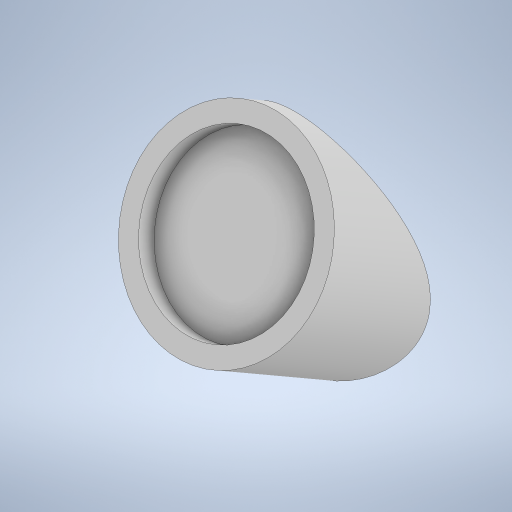
# Autodesk Inventor part: 1'' copper pipe 60 deg mount
Saved by Autodesk Inventor 2024.2 (Build 282272000, 272)
## iProperties
Created: 2024-03-22
Part Number: 1'' copper pipe 60 deg mount
Material: Generic
Document SubType Name: Modeling
Designer: ellix
Density: 1 g/cm^3
Appearance: Default
Author: ellix
Autodesk Inventor part; units mm, degrees
ref_plane "YZ Plane" through (0, 0, 0) normal (1, 0, 0) x (0, 1, 0)
ref_plane "XZ Plane" through (0, 0, 0) normal (0, 1, 0) x (-1, 0, 0)
ref_plane "XY Plane" through (0, 0, 0) normal (0, 0, 1) x (1, 0, 0)
sketch "Sketch1" plane through (0, 0, 0) normal (1, 0, 0) x (0, 1, 0)
  line L0 (22.9037, 13.0375) -> (-26.2512, 13.0375)
  line L1 (-26.2512, 13.0375) -> (-26.2512, -17.8825)
  line L2 (-26.2512, -17.8825) -> (22.9037, -17.8825)
  line L3 (22.9037, -17.8825) -> (22.9037, 13.0375)
  line L4 (-27.7512, 14.5375) -> (24.4037, 14.5375)
  line L5 (24.4037, 14.5375) -> (24.4037, -19.3825)
  line L6 (24.4037, -19.3825) -> (-27.7512, -19.3825)
  line L7 (-27.7512, -19.3825) -> (-27.7512, 14.5375)
  line L8 (14.8755, 31.453) -> (106.1225, 31.453) construction
  line L9 (5.1094, 14.5375) -> (-10.0461, 23.2875)
  line L10 (-10.0461, 23.2875) -> (-9.0461, 25.0195)
  line L11 (-9.0461, 25.0195) -> (-10.7781, 26.0195)
  line L12 (-10.7781, 26.0195) -> (-17.4073, 14.5375)
  line L13 (24.4037, -2.4225) -> (-27.7512, -2.4225)
  point P0 (0, 0)
  point P1 (22.9037, -2.4225)
  point P2 (-26.2512, -2.4225)
  dimension "d0" = 30.92
  dimension "d1" = 1.5
  dimension "d3" = 17.5
  dimension "d4" = 2
  dimension "d5" = 2
  constraints: 28 end point, 4 parallel, 3 horizontal, 3 perpendicular, 2 midpoint, 2 point on line, 3 other
  measures "d0" distance of L2.end L0.start
  measures "d1" distance between parallel lines of L0 L4
  measures "d3" distance of L9.start L9.end
  measures "d4" distance of L9.end L10.end
  measures "d5" distance of L10.end L11.end
ref_plane "Work Plane1" through (0, -10.7781, 26.0195) normal (0, -0.5, -0.8660254) x (1, 0, 0)
sketch "Sketch2" plane through (0, -10.7781, 26.0195) normal (0, -0.5, -0.8660254) x (1, 0, 0)
  line L0 (0, -19.5) -> (0, -2) projected
  circle A0 centre (0, -10.75) radius 8.75
  circle A1 centre (0, -10.75) radius 10.75
  point P0 (0, -22.3439)
  point P1 (0, 0)
  constraints: 2 vertical alignment, 1 coincident, 1 midpoint, 4 other
extrude "Extrusion1" add sketch "Sketch2" along normal blind 19 contours A0 L0 | L0 A0 | A1
extrude "Extrusion2" cut sketch "Sketch2" along normal blind 2 contours A0 L0 | L0 A0
revolve "Revolution1" add sketch "Sketch1" angle 360 about axis through (0, 24.4037, -2.4225) along (0, -1, 0) contours L0 L1 L13 L7 L4 L5 L3
sketch "Sketch3" plane through (0, 24.4037, -2.4225) normal (0, 1, 0) x (1, 0, 0)
  circle A0 centre (0, 0) radius 15.46 projected
  circle A1 centre (0, 0) radius 16.96 projected
  point P0 (0, -2.4225)
extrude "Extrusion3" cut sketch "Sketch3" against normal blind 127.25 contours A0
sketch "Sketch4" plane through (0, 0, 0) normal (1, 0, 0) x (0, 1, 0)
  line L0 (24.4037, 14.5375) -> (-27.7512, 14.5375) projected
  line L1 (7.5764, 14.5375) -> (27.5764, 14.5375)
  line L2 (27.5764, 14.5375) -> (27.5764, -29.1021)
  line L3 (27.5764, -29.1021) -> (7.5764, -29.1021)
  line L4 (7.5764, -29.1021) -> (7.5764, 14.5375)
  line L5 (-19.8823, 14.5375) -> (-31.1808, 14.5375)
  line L6 (-31.1808, 14.5375) -> (-31.1808, -26.5715)
  line L7 (-31.1808, -26.5715) -> (-19.8823, -26.5715)
  line L8 (-19.8823, -26.5715) -> (-19.8823, 14.5375)
  point P0 (0, 0)
  dimension "d21" = 20
  constraints: 16 end point, 4 parallel, 2 horizontal, 2 perpendicular, 2 point on line
  measures "d21" distance of L2.end L3.end
extrude "Extrusion4" cut sketch "Sketch4" along normal mid plane 127.25
sketch "Sketch5" plane through (0, 7.5764, -2.4225) normal (0, 1, 0) x (1, 0, 0)
  circle A0 centre (0, 0) radius 16.96 projected
  line L0 (0, 0) -> (-20.3133, -17.0449)
  line L1 (0, 0) -> (26.5172, 0) construction
  line L2 (0, 0) -> (23.4558, -19.6818)
  line L3 (0, 0) -> (30.6194, 0) construction
  arc A1 (23.4558, -19.6818) -> (-20.2121, -16.96) centre (2.837, 1.1755) ccw
  dimension "d17" = 140
  dimension "d18" = 40
  constraints: 8 end point, 2 equal length, 2 horizontal, 2 point on circle, 1 centre point, 1 point on line
  measures "d17" angle of L0 L1
  measures "d18" angle of L2 L3
extrude "Extrusion6" cut sketch "Sketch5" against normal blind 127.25 contours A0 L2 L0 | A0 L0 A1 L2 picked at (5.2916, 9.8999)
sketch "Sketch6" plane through (0, 0, 0) normal (0, 0, 1) x (1, 0, 0)
  point P0 (0, 0)
  constraints: 3 other
sketch "Sketch7" plane through (0, -1.4684, 20.6445) normal (0, 0.5, 0.8660254) x (1, 0, 0)
  circle A0 centre (0, 0) radius 10.75 projected
  circle A1 centre (0, 0) radius 22.5
  point P0 (0, 11.5939)
  dimension "d22" = 45
  constraints: 1 centre point, 1 coincident
  measures "d22" diameter of A1
extrude "Extrusion7" cut sketch "Sketch7" against normal blind 38
body "Solid1"
